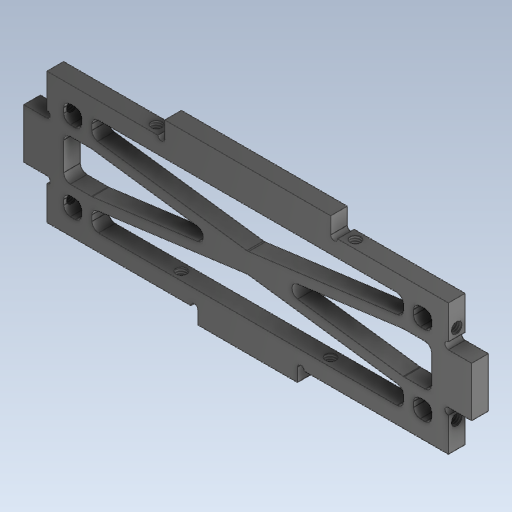
# Autodesk Inventor part: Trunk_waisit_diagonal
Saved by Autodesk Inventor 2020.4 (Build 244396000, 396)
## iProperties
Created: 2022-01-14
Part Number: Trunk_waisit_diagonal
Material: アセタール樹脂、黒
Document SubType Name: Modeling
Designer: Masato Kubotera
Density: 1.425 g/cm^3
Appearance: 滑らか - 黒
Description: POM T5
Author: Masato Kubotera
Autodesk Inventor part; units mm, degrees
ref_plane "YZ Plane" through (0, 0, 0) normal (1, 0, 0) x (0, 1, 0)
ref_plane "XZ Plane" through (0, 0, 0) normal (0, 1, 0) x (-1, 0, 0)
ref_plane "XY Plane" through (0, 0, 0) normal (0, 0, 1) x (1, 0, 0)
sketch "スケッチ1" plane through (0, 0, 0) normal (1, 0, 0) x (0, 1, 0)
  line L0 (60.5, 19.75) -> (-60.5, 19.75) construction
  line L1 (-60.5, 19.75) -> (-60.5, -19.75)
  line L2 (-60.5, -19.75) -> (60.5, -19.75) construction
  line L3 (60.5, -19.75) -> (60.5, 19.75) construction
  line L4 (60.5, 19.75) -> (-60.5, -19.75) construction
  line L5 (-60.5, 19.75) -> (60.5, -19.75) construction
  line L6 (60.5, 0) -> (-60.5, 0) construction
  line L7 (0, 19.75) -> (0, -19.75) construction
  line L8 (60.5, 7.5) -> (67.5, 7.5)
  line L9 (67.5, 7.5) -> (67.5, -7.5)
  line L10 (67.5, 0) -> (60.5, 0) construction
  arc A0 (60.5, 9.6) -> (60.5, 7.5) centre (60.5, 8.55) ccw
  line L11 (60.5, -7.5) -> (67.5, -7.5)
  arc A1 (60.5, -7.5) -> (60.5, -9.6) centre (60.5, -8.55) ccw
  line L12 (60.5, 9.6) -> (60.5, 19.75)
  line L13 (60.5, -9.6) -> (60.5, -19.75)
  line L14 (25, 19.75) -> (25, 24.75)
  line L15 (25, 24.75) -> (-25, 24.75)
  arc A2 (25, 19.75) -> (27.1, 19.75) centre (26.05, 19.75) ccw
  line L16 (27.1, 19.75) -> (60.5, 19.75)
  line L17 (-60.5, 19.75) -> (60.5, 19.75) construction
  line L18 (60.5, -19.75) -> (-60.5, -19.75) construction
  line L19 (-25, 19.75) -> (-25, 24.75)
  arc A3 (-27.1, 19.75) -> (-25, 19.75) centre (-26.05, 19.75) ccw
  line L20 (-27.1, 19.75) -> (-60.5, 19.75)
  line L21 (60.5, -19.75) -> (17.1, -19.75)
  line L22 (15, -19.75) -> (15, -23.75)
  line L23 (15, -23.75) -> (-15, -23.75)
  arc A4 (17.1, -19.75) -> (15, -19.75) centre (16.05, -19.75) ccw
  line L24 (-60.5, -19.75) -> (-17.1, -19.75)
  line L25 (-15, -19.75) -> (-15, -23.75)
  arc A5 (-15, -19.75) -> (-17.1, -19.75) centre (-16.05, -19.75) ccw
  line L26 (0, 24.75) -> (0, -23.75)
  line L27 (-55.5, -14.75) -> (55.5, -14.75) construction
  line L28 (55.5, -14.75) -> (55.5, 14.75) construction
  line L29 (55.5, 14.75) -> (-55.5, 14.75) construction
  line L30 (-55.5, 14.75) -> (-55.5, -14.75) construction
  line L31 (-55.5, -14.75) -> (55.5, 14.75) construction
  line L32 (55.5, -14.75) -> (-55.5, 14.75) construction
  line L33 (60.5, 12) -> (55.5, 12) construction
  line L34 (60.5, 10) -> (55.5, 10) construction
  line L35 (60.5, 14) -> (55.5, 14) construction
  line L36 (60.5, -12) -> (55.5, -12) construction
  line L37 (60.5, -10) -> (55.5, -10) construction
  line L38 (60.5, -14) -> (55.5, -14) construction
  line L39 (53.5, 14.75) -> (52, 14.75)
  line L40 (50, 12.75) -> (50, 11.25)
  line L41 (52, 9.25) -> (53.5, 9.25)
  line L42 (55.5, 11.25) -> (55.5, 12.75)
  line L43 (55.5, 14.75) -> (50, 9.25) construction
  line L44 (50, 14.75) -> (55.5, 9.25) construction
  arc A6 (55.5, 12.75) -> (53.5, 14.75) centre (53.5, 12.75) ccw
  arc A7 (53.5, 9.25) -> (55.5, 11.25) centre (53.5, 11.25) ccw
  arc A8 (50, 11.25) -> (52, 9.25) centre (52, 11.25) ccw
  arc A9 (52, 14.75) -> (50, 12.75) centre (52, 12.75) ccw
  line L45 (53.5, -14.75) -> (52, -14.75)
  line L46 (52, -9.25) -> (53.5, -9.25)
  line L47 (55.5, -11.25) -> (55.5, -12.75)
  arc A10 (53.5, -14.75) -> (55.5, -12.75) centre (53.5, -12.75) ccw
  arc A11 (55.5, -11.25) -> (53.5, -9.25) centre (53.5, -11.25) ccw
  arc A12 (52, -9.25) -> (50, -11.25) centre (52, -11.25) ccw
  arc A13 (50, -12.75) -> (52, -14.75) centre (52, -12.75) ccw
  line L48 (50, -12.75) -> (50, -11.25)
  line L49 (47, 12.75) -> (47, 11.0273)
  line L50 (45.2647, 9.0449) -> (0.2647, 3.0354)
  line L51 (15.0438, 1.9824) -> (46.8682, 6.2324)
  line L52 (47.133, 6.25) -> (53.5, 6.25)
  line L53 (15.0438, -1.9824) -> (46.8682, -6.2324)
  line L54 (55.5, 4.25) -> (55.5, -4.25)
  line L55 (47.133, -6.25) -> (53.5, -6.25)
  arc A14 (55.5, 4.25) -> (53.5, 6.25) centre (53.5, 4.25) ccw
  arc A15 (53.5, -6.25) -> (55.5, -4.25) centre (53.5, -4.25) ccw
  arc A16 (46.8682, -6.2324) -> (47.133, -6.25) centre (47.133, -4.25) ccw
  arc A17 (15.0438, 1.9824) -> (15.0438, -1.9824) centre (15.3086, 0) ccw
  arc A18 (47.133, 6.25) -> (46.8682, 6.2324) centre (47.133, 4.25) ccw
  line L56 (0, 14.75) -> (45, 14.75)
  line L57 (-47, 9.2766) -> (-0.2647, 3.0354)
  arc A19 (47, 12.75) -> (45, 14.75) centre (45, 12.75) ccw
  arc A20 (45.2647, 9.0449) -> (47, 11.0273) centre (45, 11.0273) ccw
  arc A21 (-0.2647, 3.0354) -> (0, 3.0178) centre (0, 5.0178) ccw
  arc A22 (0, 3.0178) -> (0.2647, 3.0354) centre (0, 5.0178) ccw
  line L58 (45.2647, -9.0449) -> (0.2647, -3.0354)
  line L59 (0, -14.75) -> (45, -14.75)
  arc A23 (45, -14.75) -> (47, -12.75) centre (45, -12.75) ccw
  arc A24 (47, -11.0273) -> (45.2647, -9.0449) centre (45, -11.0273) ccw
  arc A25 (0.2647, -3.0354) -> (0, -3.0178) centre (0, -5.0178) ccw
  line L60 (47, -12.75) -> (47, -11.0273)
  point P0 (0, 0)
  point P1 (52.75, 12)
  point P2 (47, 9.2766)
  point P3 (0, 3)
  point P4 (0.1994, 0)
  point P5 (47, 6.25)
  point P6 (55.5, 6.25)
  point P7 (55.5, 0)
  point P8 (47, -6.25)
  point P9 (55.5, -6.25)
  point P10 (0, -3.0178)
  dimension "d0" = 121
  dimension "d1" = 39.5
  dimension "d2" = 1.05
  dimension "d3" = 7
  dimension "d4" = 15
  dimension "d5" = 0
  dimension "d6" = 1.05
  dimension "d7" = 5
  dimension "d8" = 50
  dimension "d9" = 1.05
  dimension "d10" = 4
  dimension "d11" = 30
  dimension "d12" = 5
  dimension "d13" = 5
  dimension "d14" = 4
  dimension "d15" = 24
  dimension "d16" = 2
  dimension "d17" = 5.5
  dimension "d20" = 3
  dimension "d21" = 5.5
  dimension "d23" = 3
  dimension "d24" = 2
  dimension "d25" = 3
  dimension "d26" = 3
  dimension "d27" = 2
  constraints: 122 end point, 52 point on circle, 47 symmetric about line, 45 point on line, 26 centre point, 26 tangent, 15 midpoint, 12 perpendicular, 9 equal radius, 7 collinear, 7 parallel, 4 horizontal, 4 vertical, 10 other
  measures "d0" distance of L2.end L1.end
  measures "d1" distance of L1.end L0.end
  measures "d2" radius of A0
  measures "d3" distance of L8.start L8.end
  measures "d4" distance of L8.end L9.end
  measures "d5" distance between parallel lines of L6 L10
  measures "d6" radius of A2
  measures "d7" distance of L14.end L14.start
  measures "d8" distance of L14.end L15.end
  measures "d9" radius of A4
  measures "d10" distance of L22.start L22.end
  measures "d11" distance of L22.end L23.end
  measures "d12" horizontal distance of L0.start L28.end
  measures "d13" horizontal distance of L28.end L0.start
  measures "d14" distance of L34.end L35.end
  measures "d15" distance of L36.start L33.start
  measures "d16" radius of A6
  measures "d17" distance of L44.start L43.end
  measures "d20" distance between parallel lines of L51 L50
  measures "d21" distance of L28.end L44.start
  measures "d23" distance between parallel lines of L52 L41
  measures "d24" radius of A14
  measures "d25" distance of point (0, 0) point (0, 3)
  measures "d26" distance between parallel lines of L49 L40
  measures "d27" radius of A19
extrude "押し出し1" add sketch "スケッチ1" along normal blind 5 contours L15 L14 A2 L16 L12 A0 L8 L9 L11 A1 L13 L21 A4 L22 L23 L26 L59 A23 L60 A24 L58 A25 A22 L50 A20 L49 A19 L56
sketch "スケッチ2" plane through (0, 60.5, 19.75) normal (0, 1, 0) x (1, 0, 0)
  line L0 (0, 39.5) -> (5, 39.5) projected
  line L1 (2.5, 39.5) -> (2.5, 0)
  line L2 (0, 0) -> (5, 0) projected
  line L3 (0, 19.75) -> (5, 19.75)
  line L4 (5, 27.25) -> (5, 12.25) projected
  point P0 (2.5, 7.75)
  point P1 (2.5, 31.75)
  dimension "d30" = 24
  constraints: 4 end point, 3 midpoint, 1 point on line, 1 symmetric about line
  measures "d30" distance of point (2.5, 7.75) point (2.5, 31.75)
hole "穴1" at (2.5, 60.5, 12) at (2.5, 60.5, -12) direction (0, -1, 0) diameter 3.242 depth 5 tip angle 118 thread size "M4x0.7" class "6H" standard "ISO Metric profile"
sketch "スケッチ3" plane through (0, 27.1, 19.75) normal (0, 0, 1) x (1, 0, 0)
  line L0 (0.879, 33.4) -> (4.121, 33.4) projected
  line L1 (2.5, 33.4) -> (2.5, -27.1)
  line L2 (0, -27.1) -> (5, -27.1) projected
  point P0 (2.5, 2.9)
  dimension "d38" = 30
  constraints: 2 end point, 2 midpoint, 1 point on line
  measures "d38" distance from line of L2 point (2.5, 2.9)
hole "穴2" at (2.5, 30, 19.75) direction (0, 0, -1) diameter 3.242 depth 5 tip angle 118 thread size "M4x0.7" class "6H" standard "ISO Metric profile"
sketch "スケッチ4" plane through (0, 17.1, -19.75) normal (0, 0, -1) x (-1, 0, 0)
  line L0 (0, -17.1) -> (-5, -17.1) projected
  line L1 (-2.5, -17.1) -> (-2.5, 43.4)
  line L2 (-4.121, 43.4) -> (-0.879, 43.4) projected
  point P0 (-2.5, 5.4)
  dimension "d46" = 22.5
  constraints: 2 end point, 2 midpoint, 1 point on line
  measures "d46" distance from line of point (-2.5, 5.4) L0
hole "穴3" at (2.5, 22.5, -19.75) direction (0, 0, 1) diameter 3.242 depth 5 tip angle 118 thread size "M4x0.7" class "6H" standard "ISO Metric profile"
mirror "ミラー1" about plane through (0, 0, 24.75) normal (0, -1, 0)
equation "\"d6\" = d2"
equation "\"d9\" = d2"
equation "\"d13\" = d12"
equation "\"d17\" = -2 * d12 + d1 - d15"
equation "\"d21\" = d17"
